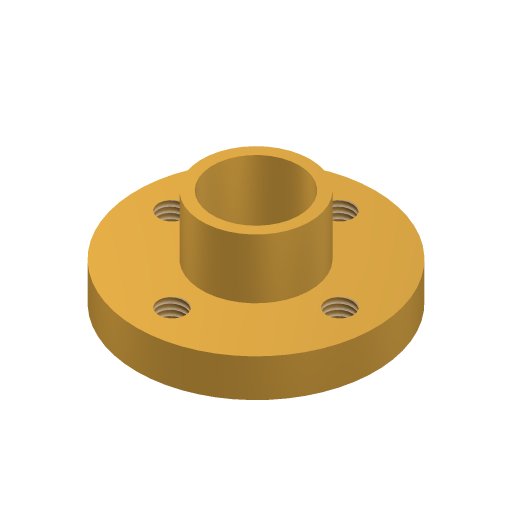
# Autodesk Inventor part: Z Axis Nut
Saved by Autodesk Inventor 2023.2 (Build 272271000, 271)
## iProperties
Created: 2020-05-09
Part Number: Z Axis Nut
Material: Brass, Soft Yellow
Document SubType Name: Modeling
Designer: Remo
Mass: 10.8922 g
Surface Area: 14.556 cm^2
Volume: 1.28597 cm^3
Density: 8.47 g/cm^3
Appearance: Brass - Satin
Author: Remo
Autodesk Inventor part; units mm, degrees
ref_plane "YZ Plane" through (0, 0, 0) normal (1, 0, 0) x (0, 1, 0)
ref_plane "XZ Plane" through (0, 0, 0) normal (0, 1, 0) x (-1, 0, 0)
ref_plane "XY Plane" through (0, 0, 0) normal (0, 0, 1) x (1, 0, 0)
sketch "Sketch1" plane through (0, 0, 0) normal (1, 0, 0) x (0, 1, 0)
  line L0 (4, -10.5) -> (4, 0)
  line L1 (0, 0) -> (0, -10.5)
  line L2 (4, -10.5) -> (5, -10.5)
  line L3 (5, -10.5) -> (5, -9)
  line L4 (5, -9) -> (11, -9)
  line L5 (11, -9) -> (11, -5.5)
  line L6 (11, -5.5) -> (5, -5.5)
  line L7 (5, -5.5) -> (5, 0)
  line L8 (5, 0) -> (4, 0)
  dimension "d0" = 10.5
  dimension "d1" = 4
  dimension "d2" = 5
  dimension "d3" = 5
  dimension "d4" = 3.5
  dimension "d10" = 11
  constraints: 18 end point, 5 perpendicular, 2 horizontal alignment, 2 point on line, 2 vertical, 1 horizontal
  measures "d0" distance of L1.start L1.end
  measures "d1" distance between parallel lines of L1 L0
  measures "d2" distance between parallel lines of L1 L3
  measures "d3" distance between parallel lines of L2 L6
  measures "d4" distance of L4.end L5.end
  measures "d10" distance between parallel lines of L1 L5
revolve "Revolution1" add sketch "Sketch1" angle 360 about axis through (0, 0, 0) along (0, 0, -1)
sketch "Sketch2" plane through (0, 0, -5.5) normal (0, 0, 1) x (1, 0, 0)
  point P0 (0, 0)
  point P1 (0, 7.75)
  point P2 (-7.75, 0)
  point P3 (0, -7.75)
  point P4 (7.75, 0)
  dimension "d6" = 15.5
  dimension "d7" = 7.75
  dimension "d8" = 15.5
  dimension "d9" = 7.75
  constraints: 1 horizontal alignment, 1 vertical alignment
  measures "d6" distance of point (0, -7.75) point (0, 7.75)
  measures "d7" distance of point (0, 7.75) point (0, 0)
  measures "d8" distance of point (-7.75, 0) point (7.75, 0)
  measures "d9" distance of point (-7.75, 0) point (0, 0)
hole "Hole1" at (0, 7.75, -5.5) at (-7.75, 0, -5.5) at (0, -7.75, -5.5) at (7.75, 0, -5.5) direction (0, 0, -1) diameter 2.459 end through all thread size "M3x0.5" class "6H" standard "ISO Metric profile"
equation "\"d7\" = 0.5 * d6"
equation "\"d9\" = 0.5 * d8"
body "Solid1"
